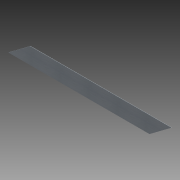
# Autodesk Inventor part: Duct_Inner_Template
Saved by Autodesk Inventor 2011 SP1 (Build 150282100, 282)
## iProperties
Created: 2011-06-12
Part Number: Duct_Inner_Template
Document SubType Name: Modeling
Designer: Andrew G. Meyer
Density: 1 g/cm^3
Mass: 79.032 g
Surface Area: 1020.45 cm^2
Volume: 79.032 cm^3
Author: Andrew G. Meyer
Autodesk Inventor part; units mm, degrees
ref_plane "YZ Plane" through (0, 0, 0) normal (1, 0, 0) x (0, 1, 0)
ref_plane "XZ Plane" through (0, 0, 0) normal (0, 1, 0) x (-1, 0, 0)
ref_plane "XY Plane" through (0, 0, 0) normal (0, 0, 1) x (1, 0, 0)
sketch "Sketch1" plane through (0, 0, 0) normal (0, 0, 1) x (1, 0, 0)
  line L0 (-384.3704, -35.5844) -> (-282.7704, 40.6156)
  line L1 (-282.7704, 40.6156) -> (370.5625, 40.6156)
  line L2 (370.5625, 40.6156) -> (268.9625, -35.5844)
  line L3 (268.9625, -35.5844) -> (-384.3704, -35.5844)
  point P0 (0, 0)
  dimension "d0" = 653.3329
  dimension "d1" = 76.2
  dimension "d2" = 101.6
  constraints: 8 end point, 3 parallel, 1 horizontal, 1 point on line
  measures "d0" distance of L0.end L1.end
  measures "d1" distance between parallel lines of L3 L1
  measures "d2" horizontal distance of L0.start L0.end
extrude "Extrusion1" add sketch "Sketch1" along normal blind 1.5875
body "Solid1"
